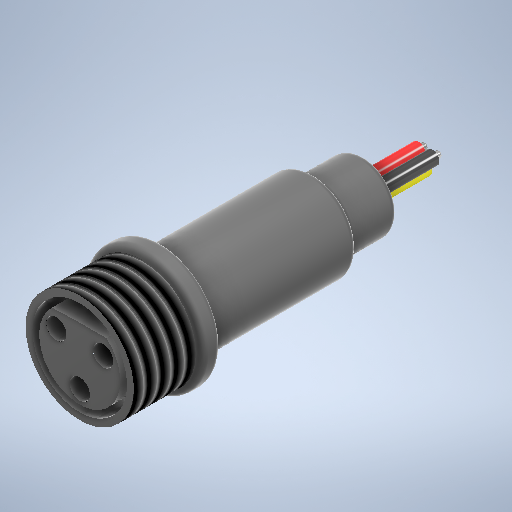
# Autodesk Inventor part: 12vplug
Saved by Autodesk Inventor 2025 (Build 290162000, 162)
## iProperties
Created: 2024-08-10
Part Number: 12vplug
Material: Generic
Document SubType Name: Modeling
Designer: ethan
Density: 1 g/cm^3
Appearance: Default
Author: ethan
Autodesk Inventor part; units mm, degrees
ref_plane "YZ Plane" through (0, 0, 0) normal (1, 0, 0) x (0, 1, 0)
ref_plane "XZ Plane" through (0, 0, 0) normal (0, 1, 0) x (-1, 0, 0)
ref_plane "XY Plane" through (0, 0, 0) normal (0, 0, 1) x (1, 0, 0)
sketch "Sketch1" plane through (0, 0, 0) normal (0, 0, 1) x (1, 0, 0)
  circle A0 centre (0, 0) radius 6.5
  dimension "d0" = 13
  constraints: 1 centre point, 1 coincident
  measures "d0" diameter of A0
extrude "Extrusion1" add sketch "Sketch1" along normal blind 22.5
sketch "Sketch2" plane through (0, 0, 22.5) normal (0, 0, 1) x (1, 0, 0)
  circle A0 centre (0, 0) radius 5
  dimension "d3" = 10
  constraints: 1 centre point, 1 coincident
  measures "d3" diameter of A0
extrude "Extrusion2" add sketch "Sketch2" along normal blind 7.5
fillet "Fillet1" radius 1 3 edges at (-6.5, 0, 22.5) (-5, 0, 30) (-5, 0, 22.5)
sketch "Sketch3" plane through (0, 0, 0) normal (0, 0, -1) x (-1, 0, 0)
  circle A0 centre (0, 0) radius 8.9
  dimension "d7" = 17.8
  constraints: 1 centre point, 1 coincident
  measures "d7" diameter of A0
extrude "Extrusion3" add sketch "Sketch3" along normal blind 3
sketch "Sketch4" plane through (0, 0, -3) normal (0, 0, -1) x (-1, 0, 0)
  circle A0 centre (0, 0) radius 8
  dimension "d10" = 16
  constraints: 1 centre point, 1 coincident
  measures "d10" diameter of A0
extrude "Extrusion4" add sketch "Sketch4" along normal blind 9.2
fillet "Fillet2" radius 1 2 edges at (8.9, 0, 0) (8.9, 0, -3)
thread "Thread1" size "M16x2" class "6g" standard "ANSI Metric M Profile" full length
sketch "Sketch5" plane through (0, 0, -12.2) normal (0, 0, -1) x (-1, 0, 0)
  circle A0 centre (0, 0) radius 4 construction
  circle A1 centre (0, 4) radius 1.5
  circle A2 centre (-3.4641, -2) radius 1.5
  circle A3 centre (3.4641, -2) radius 1.5
  dimension "d16" = 8
  dimension "d17" = 3
  dimension "d20" = 360
  constraints: 3 centre point, 1 coincident, 1 vertical alignment, 9 other
  measures "d17" diameter of A1
extrude "Extrusion5" cut sketch "Sketch5" against normal blind 9.2
sketch "Sketch6" plane through (0, 0, 30) normal (0, 0, 1) x (1, 0, 0)
  line L0 (0, 0) -> (0, 1.2)
  circle A0 centre (0, 1.2) radius 1
  circle A1 centre (-1.0392, -0.6) radius 1
  circle A2 centre (1.0392, -0.6) radius 1
  dimension "d24" = 1.2
  dimension "d25" = 2
  dimension "d28" = 360
  constraints: 3 centre point, 2 end point, 1 coincident, 1 vertical, 7 other
  measures "d24" distance of L0.start L0.end
  measures "d25" diameter of A0
extrude "Extrusion6" add sketch "Sketch6" along normal blind 10
sketch "Sketch7" plane through (0, 1.2, 40) normal (0, 0, 1) x (1, 0, 0)
  circle A0 centre (0, 0) radius 1 construction
  circle A1 centre (1.0392, -1.8) radius 1 construction
  circle A2 centre (-1.0392, -1.8) radius 1 construction
  circle A3 centre (0, 0) radius 0.5
  circle A4 centre (1.0392, -1.8) radius 0.5
  circle A5 centre (-1.0392, -1.8) radius 0.5
  circle A6 centre (-1.0392, -1.8) radius 1
  circle A7 centre (1.0392, -1.8) radius 1
  circle A8 centre (0, 0) radius 1
  point P0 (0, -1.2)
  dimension "d32" = 1
  dimension "d33" = 1
  dimension "d34" = 1
  constraints: 6 centre point, 6 coincident, 3 concentric
  measures "d32" diameter of A3
  measures "d33" diameter of A4
  measures "d34" diameter of A5
extrude "Extrusion7" cut sketch "Sketch7" against normal blind 1
fillet "Fillet3" radius 0.25 3 edges at (-0.5, 1.2, 40) (-1.5392, -0.6, 40) (0.5392, -0.6, 40)
sketch "Sketch8" plane through (0, 0, -12.2) normal (0, 0, -1) x (-1, 0, 0)
  arc A0 (4.0943, -4.3859) -> (-3.9686, -4.5) centre (0, 0) ccw
  circle A1 centre (0, 0) radius 7
  line L0 (0, -4.5) -> (-3.9686, -4.5)
  line L1 (0, -4.5) -> (4.0943, -4.3859)
  dimension "d38" = 12
  dimension "d39" = 14
  constraints: 4 end point, 2 centre point, 2 coincident, 2 point on circle
  measures "d38" diameter of A0
  measures "d39" diameter of A1
extrude "Extrusion8" cut sketch "Sketch8" against normal blind 6
equation "\"d35\" = d34"
body "Solid1"
